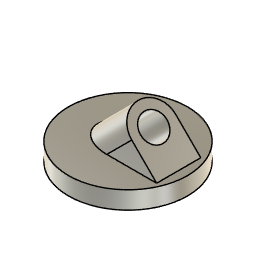
17 (Autodesk Fusion 360 design; units mm, degrees)
Autodesk Fusion 360 part; units mm, degrees
sketch "草图1" plane through (0, 0, 0) normal (0, 0, 1) x (1, 0, 0)
  circle A0 centre (0, 0) radius 27
  circle A1 centre (0, 0) radius 20
  dimension "d1" = 54
  dimension "d2" = 40
  constraint coincident A0.centre A1.centre
  measures "d1" diameter of A0
  measures "d2" diameter of A1
extrude "拉伸1" add sketch "草图1" against normal blind 8
extrude "拉伸2" add sketch "草图1" against normal blind 3 contours A1
sketch "草图2" plane through (0, 0, 0) normal (0, 0, 1) x (-1, 0, 0)
  circle A0 centre (0, 0) radius 27
  line L0 (-23, -10) -> (-23, 10)
  line L1 (30, 0) -> (-47, 0) construction
  dimension "d7" = 20
  dimension "d8" = 23
  constraint vertical L0
  constraint horizontal L1
  constraint symmetric L0.start L0.end L1
  measures "d7" distance of L0.start L0.end
  measures "d8" distance of A0.centre L0
ref_plane "工作平面1" through (23, 0, 0) normal (0.707107, 0, 0.707107) x (0, -1, 0)
sketch "草图3" plane through (11.5, 0, 11.5) normal (0.707107, 0, 0.707107) x (0, -1, 0)
  circle A0 centre (0, 0.2635) radius 6
  line L0 (10, 0.2635) -> (10, 16.2635)
  line L1 (10, 16.2635) -> (-10, 16.2635)
  line L2 (-10, 16.2635) -> (-10, 0.2635)
  line L3 (0, 0) -> (0, 19) construction
  arc A1 (-10, 0.2635) -> (10, 0.2635) centre (0, 0.2635) ccw
  dimension "d10" = 10
  dimension "d11" = 12
  dimension "d12" = 16
  constraint concentric A0 A1
  constraint vertical L0
  constraint horizontal L1
  constraint vertical L2
  constraint coincident L3.start origin
  constraint collinear L3.start A0.centre L3.end
  constraint tangent L0 A1
  constraint tangent L2 A1
  measures "d10" radius of A1
  measures "d11" diameter of A0
  measures "d12" distance of L2.end L1.end
extrude "拉伸3" add sketch "草图3" along normal up to surface end surface through (0, 0, -3) normal (0, 0, -1) offset 0
extrude "拉伸4" cut sketch "草图3" along normal up to surface contours A0 end surface through (0, 0, -3) normal (0, 0, -1) offset 0
